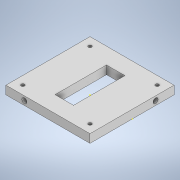
# Autodesk Inventor part: platforma wriertnicza
Saved by Autodesk Inventor 2020 (Build 240168000, 168)
## iProperties
Created: 2023-01-05
Part Number: platforma wriertnicza
Material: Ogólny
Document SubType Name: Modeling
Designer: User
Density: 1 g/cm^3
Appearance: Domyślna
Author: User
Autodesk Inventor part; units mm, degrees
ref_plane "YZ Plane" through (0, 0, 0) normal (1, 0, 0) x (0, 1, 0)
ref_plane "XZ Plane" through (0, 0, 0) normal (0, 1, 0) x (-1, 0, 0)
ref_plane "XY Plane" through (0, 0, 0) normal (0, 0, 1) x (1, 0, 0)
sketch "Szkic1" plane through (0, 0, 0) normal (0, 1, 0) x (-1, 0, 0)
  line L0 (25, 25) -> (-25, 25)
  line L1 (-25, 25) -> (-25, -25)
  line L2 (-25, -25) -> (25, -25)
  line L3 (25, -25) -> (25, 25)
  line L4 (0, 25) -> (0, -25)
  line L5 (25, 0) -> (-25, 0)
  circle A0 centre (20, -20) radius 2.5
  circle A1 centre (20, 20) radius 2.5
  circle A2 centre (-20, -20) radius 2.5
  circle A3 centre (-20, 20) radius 2.5
  line L6 (-5.5, 15.3) -> (5.5, 15.3)
  line L7 (5.5, 15.3) -> (5.5, -15.3)
  line L8 (5.5, -15.3) -> (-5.5, -15.3)
  line L9 (-5.5, -15.3) -> (-5.5, 15.3)
  point P0 (0, 0)
  point P1 (0, 0)
  dimension "d0" = 50
  dimension "d1" = 50
  dimension "d2" = 25
  dimension "d3" = 25
  dimension "d4" = 5
  dimension "d5" = 20
  dimension "d6" = 20
  dimension "d69" = 11
  dimension "d70" = 30.6
  constraints: 20 end point, 5 midpoint, 4 centre point, 4 parallel, 4 perpendicular, 2 horizontal, 1 coincident, 1 symmetric about line, 5 other
  measures "d0" distance of L2.end L0.start
  measures "d1" distance of L1.end L2.end
  measures "d2" distance between parallel lines of L3 L4
  measures "d3" distance between parallel lines of L2 L5
  measures "d4" diameter of A0
  measures "d5" distance from line of A0.centre L4
  measures "d6" distance from line of A0.centre L5
  measures "d69" distance of L6.start L6.end
  measures "d70" distance of L8.end L6.start
sketch "Szkic2" plane through (0, 0, 0) normal (0, 1, 0) x (-1, 0, 0)
  point P0 (0, 0)
extrude "Wyciągnięcie proste1" add sketch "Szkic1" along normal blind 5 contours L3 L5 L7 L6 L4 L0 | L4 L6 L9 L5 L1 L0 | L3 L2 L4 L8 L7 L5 | L5 L9 L8 L4 L2 L1 | A0 | A1 | A2 | A3
sketch "Szkic3" plane through (0, 0, 0) normal (0, -1, 0) x (1, 0, 0)
  circle A0 centre (-20, -20) radius 2.5
  line L0 (0, 29.2243) -> (0, -29.2243)
  line L1 (55.447, 0) -> (-42.023, 0)
  circle A1 centre (20, -20) radius 2.5
  circle A2 centre (-20, 20) radius 2.5
  circle A3 centre (20, 20) radius 2.5
  point P0 (0, 0)
  point P1 (0, 0)
  dimension "d9" = 5
  dimension "d10" = 20
  dimension "d11" = 20
  constraints: 4 centre point, 4 end point, 1 coincident, 1 horizontal, 1 midpoint, 1 perpendicular, 1 point on line, 1 vertical, 3 other
  measures "d9" diameter of A0
  measures "d10" distance from line of A0.centre L1
  measures "d11" distance from line of A0.centre L0
hole "Otwór1" at (20, 0, -20) at (-20, 0, -20) at (-20, 0, 20) at (20, 0, 20) direction (0, 1, 0) diameter 5 depth 2.5
sketch "Szkic4" plane through (0, 5, 0) normal (0, 1, 0) x (1, 0, 0)
  line L0 (53.1876, 0) -> (-53.1876, 0)
  line L1 (0, 32.3787) -> (0, -30.0481)
  circle A0 centre (20, -20) radius 2.5 projected
  circle A1 centre (20, -20) radius 2.5
  circle A2 centre (-20, -20) radius 2.5
  circle A3 centre (20, 20) radius 2.5 projected
  circle A4 centre (20, 20) radius 2.5
  circle A5 centre (-20, 20) radius 2.5 projected
  circle A6 centre (-20, 20) radius 2.5
  point P0 (0, 0)
  point P1 (0, 0)
  constraints: 4 centre point, 4 end point, 3 coincident, 2 midpoint, 2 point on line, 1 horizontal, 1 vertical, 2 other
hole "Otwór2" at (-20, 5, -20) at (20, 5, -20) at (20, 5, 20) at (-20, 5, 20) direction (0, -1, 0) diameter 2 depth 2.5
sketch "Szkic5" plane through (25, 0, 25) normal (1, 0, 0) x (0, 0, -1)
  circle A0 centre (39, 2.5) radius 1.5
  line L0 (0, 0) -> (50, 0) projected
  line L1 (50, 0) -> (50, 5) projected
  point P0 (25, 0)
  dimension "d26" = 3
  dimension "d27" = 2.5
  dimension "d28" = 11
  constraints: 1 centre point
  measures "d26" diameter of A0
  measures "d27" distance from line of L0 A0.centre
  measures "d28" distance from line of L1 A0.centre
sketch "Szkic6" plane through (-25, 0, -25) normal (-1, 0, 0) x (0, 0, 1)
  circle A0 centre (11, 2.5) radius 1.5
  line L0 (0, 0) -> (0, 5) projected
  line L1 (0, 0) -> (50, 0) projected
  point P0 (25, 0)
  dimension "d29" = 3
  dimension "d30" = 11
  dimension "d31" = 2.5
  constraints: 1 centre point
  measures "d29" diameter of A0
  measures "d30" distance from line of L0 A0.centre
  measures "d31" distance from line of L1 A0.centre
sketch "Szkic7" plane through (-25, 0, 25) normal (0, 0, 1) x (1, 0, 0)
  circle A0 centre (11, 2.5) radius 1.5
  line L0 (0, 0) -> (0, 5) projected
  line L1 (0, 0) -> (50, 0) projected
  point P0 (25, 0)
  dimension "d32" = 3
  dimension "d33" = 11
  dimension "d34" = 2.5
  constraints: 1 centre point
  measures "d32" diameter of A0
  measures "d33" distance from line of L0 A0.centre
  measures "d34" distance from line of L1 A0.centre
hole "Otwór3" at (-14, 2.5, 25) direction (0, 0, -1) diameter 3 depth 3
hole "Otwór4" at (-25, 2.5, -14) direction (1, 0, 0) diameter 3 depth 3
hole "Otwór5" at (25, 2.5, -14) direction (-1, 0, 0) diameter 3 depth 3
sketch "Szkic8" plane through (25, 0, -25) normal (0, 0, -1) x (-1, 0, 0)
  circle A0 centre (6.25, 2.5) radius 0.5
  line L0 (0, 0) -> (0, 5) projected
  line L1 (0, 0) -> (50, 0) projected
  circle A1 centre (43.75, 2.5) radius 0.5
  line L2 (50, 0) -> (50, 5) projected
  point P0 (25, 0)
  dimension "d56" = 6.25
  dimension "d57" = 1
  dimension "d58" = 2.5
  dimension "d59" = 1
  dimension "d60" = 6.25
  dimension "d61" = 2.5
  constraints: 2 centre point
  measures "d56" distance from line of L0 A0.centre
  measures "d57" diameter of A0
  measures "d58" distance from line of L1 A0.centre
  measures "d59" diameter of A1
  measures "d60" distance from line of L2 A1.centre
  measures "d61" distance from line of L1 A1.centre
hole "Otwór6" at (18.75, 2.5, -25) at (-18.75, 2.5, -25) direction (0, 0, 1) diameter 1 depth 2.5
sketch "Szkic9" plane through (25, 0, 25) normal (1, 0, 0) x (0, 0, -1)
  point P0 (25, 0)
